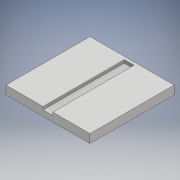
# Autodesk Inventor part: Voorplaat
Saved by Autodesk Inventor 2018.3 (Build 223284000, 284)
## iProperties
Created: 2020-11-10
Part Number: Voorplaat
Material: Generic
Document SubType Name: Modeling
Designer: daanv
Density: 1 g/cm^3
Appearance: Default
Author: daanv
Autodesk Inventor part; units mm, degrees
ref_plane "YZ Plane" through (0, 0, 0) normal (1, 0, 0) x (0, 1, 0)
ref_plane "XZ Plane" through (0, 0, 0) normal (0, 1, 0) x (-1, 0, 0)
ref_plane "XY Plane" through (0, 0, 0) normal (0, 0, 1) x (1, 0, 0)
sketch "Sketch1" plane through (0, 0, 0) normal (0, 0, 1) x (1, 0, 0)
  line L0 (0, 0) -> (14.7, 0)
  line L1 (14.7, 0) -> (14.7, 14.7)
  line L2 (14.7, 14.7) -> (0, 14.7)
  line L3 (0, 14.7) -> (0, 0)
  dimension "d0" = 14.7
  dimension "d1" = 14.7
  constraints: 8 end point, 2 parallel, 1 horizontal, 1 perpendicular
  measures "d0" distance of L2.end L1.end
  measures "d1" distance of L1.end L0.end
extrude "Extrusion1" add sketch "Sketch1" along normal blind 1.5
sketch "Sketch2" plane through (0, 0, 1.5) normal (0, 0, 1) x (1, 0, 0)
  line L0 (0, 0) -> (14.7, 0) projected
  line L1 (14.7, 14.7) -> (0, 14.7) projected
  line L2 (8.2, 14.7) -> (8.2, 0)
  line L3 (6.5, 14.7) -> (6.5, 0)
  dimension "d6" = 1.7
  dimension "d7" = 6.5
  constraints: 4 end point, 4 point on line, 2 perpendicular
  measures "d6" distance of L2.start L3.start
  measures "d7" distance of L1.end L3.start
extrude "Extrusion2" cut sketch "Sketch2" against normal blind 0.5
sketch "Sketch3" plane through (0, 0, 1) normal (0, 0, 1) x (1, 0, 0)
  line L0 (8.2, 14.7) -> (8.2, 0) projected
  line L1 (6.5, 14.7) -> (8.2, 14.7)
  line L2 (8.2, 14.7) -> (8.2, 14.2)
  line L3 (8.2, 14.2) -> (6.5, 14.2)
  line L4 (6.5, 14.2) -> (6.5, 14.7)
  point P0 (0, 0)
  dimension "d8" = 0.5
  constraints: 8 end point, 2 parallel, 1 horizontal, 1 perpendicular, 1 point on line
  measures "d8" distance of L1.end L2.end
extrude "Extrusion3" add sketch "Sketch3" along normal blind 0.5
body "Solid1"
